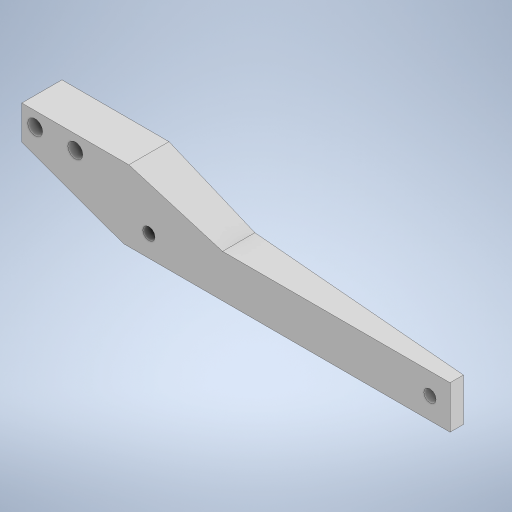
# Autodesk Inventor part: Fan_side_mount
Saved by Autodesk Inventor 2023 (Build 270158000, 158)
## iProperties
Created: 2023-08-19
Part Number: Fan_side_mount
Material: Generic
Document SubType Name: Modeling
Designer: plebbb
Density: 1 g/cm^3
Appearance: Default
Author: plebbb
Autodesk Inventor part; units mm, degrees
ref_plane "YZ Plane" through (0, 0, 0) normal (1, 0, 0) x (0, 1, 0)
ref_plane "XZ Plane" through (0, 0, 0) normal (0, 1, 0) x (-1, 0, 0)
ref_plane "XY Plane" through (0, 0, 0) normal (0, 0, 1) x (1, 0, 0)
sketch "Sketch1" plane through (0, 0, 0) normal (0, 1, 0) x (-1, 0, 0)
  line L0 (0, 0) -> (-40, 0)
  line L1 (-40, 0) -> (-160, 10)
  line L2 (-160, 10) -> (-160, 15)
  line L3 (-160, 15) -> (0, 15)
  line L4 (0, 15) -> (0, 0)
  point P0 (-160, 12.5)
  dimension "d0" = 15
  dimension "d1" = 40
  dimension "d2" = 5
  dimension "d3" = 120
  constraints: 10 end point, 3 perpendicular, 1 horizontal, 1 midpoint
  measures "d0" distance of L3.end L0.start
  measures "d1" distance of L0.start L0.end
  measures "d2" distance of L1.end L2.end
  measures "d3" horizontal distance of L0.end point (-160, 12.5)
extrude "Extrusion1" add sketch "Sketch1" along normal blind 16
sketch "Sketch2" plane through (0, 0, 15) normal (0, 0, 1) x (1, 0, 0)
  circle A0 centre (152.5, 8) radius 2.286
  circle A1 centre (47.5, 8) radius 2.286
  line L0 (160, 0) -> (160, 16) projected
  point P0 (0, 0)
  point P1 (160, 8)
  dimension "d6" = 4.572
  dimension "d7" = 7.5
  dimension "d8" = 105
  constraints: 2 centre point, 2 horizontal alignment, 1 equal radius, 1 midpoint
  measures "d6" diameter of A0
  measures "d7" distance of point (160, 8) A0.centre
  measures "d8" distance of A0.centre A1.centre
extrude "Extrusion2" cut sketch "Sketch2" against normal blind 20
sketch "Sketch3" plane through (40, 0, 0) normal (0, 0, -1) x (-1, 0, 0)
  circle A0 centre (-112.5, 8) radius 2.286 projected
  circle A1 centre (-112.5, 8) radius 6
  circle A2 centre (-7.5, 8) radius 2.286 projected
  circle A3 centre (-7.5, 8) radius 6
  point P0 (40, 0)
  dimension "d11" = 12
  constraints: 2 centre point, 2 coincident, 1 equal radius
  measures "d11" diameter of A1
extrude "Extrusion3" cut sketch "Sketch3" against normal up to surface (10 mm away)
sketch "Sketch4" plane through (40, 0, 0) normal (0, 0, -1) x (-1, 0, 0)
  line L0 (40, 0) -> (40, 16) projected
  line L1 (40, 0) -> (40, 16) projected
  line L2 (40, 16) -> (40, 26.5)
  line L3 (40, 26.5) -> (0, 26.5)
  line L4 (0, 26.5) -> (0, 16)
  line L5 (0, 0) -> (0, 16) projected
  line L6 (0, 0) -> (40, 0) projected
  line L7 (40, 0) -> (40, 16) projected
  line L8 (0, 16) -> (40, 16) projected
  point P0 (40, 8)
  dimension "d14" = 18.5
  constraints: 6 end point, 1 horizontal, 1 midpoint, 1 point on line, 1 vertical
  measures "d14" distance of L2.end point (40, 8)
extrude "Extrusion4" add sketch "Sketch4" against normal up to surface (15 mm away) contours L8 L4 L3 L2
sketch "Sketch5" plane through (40, 0, 0) normal (0, 0, -1) x (-1, 0, 0)
  line L0 (40, 0) -> (-120, 0) projected
  line L1 (2, 0) -> (2, 13.8)
  line L2 (2, 13.8) -> (40, 13.8)
  line L3 (40, 0) -> (40, 26.5) projected
  line L4 (40, 26.5) -> (0, 26.5) projected
  line L5 (0, 26.5) -> (0, 16) projected
  dimension "d17" = 12.7
  dimension "d18" = 2
  constraints: 4 end point, 2 perpendicular, 2 point on line
  measures "d17" distance between parallel lines of L4 L2
  measures "d18" distance between parallel lines of L5 L1
extrude "Extrusion5" cut sketch "Sketch5" against normal through all
sketch "Sketch6" plane through (40, 0, 15) normal (0, 0, -1) x (-1, 0, 0)
  line L0 (40, 13.8) -> (40, 26.5) projected
  line L1 (2, 13.8) -> (2, 0) projected
  line L2 (40, 13.8) -> (2, 0)
  line L3 (2, 13.8) -> (40, 13.8) projected
  point P0 (40, 0)
  constraints: 2 end point
extrude "Extrusion6" add sketch "Sketch6" along normal blind 3
chamfer "Chamfer1" distance 3 angle 45 3 edges at (38, 6.9, 12) (38, 13.8, 6) (19, 13.8, 12)
sketch "Sketch7" plane through (160, 0, 15) normal (0, 0, 1) x (1, 0, 0)
  line L0 (-120, 26.5) -> (-120, 16) projected
  line L1 (-120, 26.5) -> (-85, 16)
  line L2 (-120, 16) -> (0, 16) projected
  point P0 (-160, 0)
  dimension "d29" = 35
  constraints: 2 end point, 1 point on line
  measures "d29" horizontal distance of L0.start L1.end
extrude "Extrusion7" add sketch "Sketch7" against normal up to surface surface through (160, 0, 10) normal (0.0830455, 0, -0.9965458)
sketch "Sketch9" plane through (160, 0, 15) normal (0, 0, 1) x (1, 0, 0)
  circle A0 centre (-140, 21.15) radius 2.794
  circle A1 centre (-155, 21.15) radius 2.794
  line L0 (-160, 13.8) -> (-160, 26.5) projected
  point P0 (-160, 0)
  point P1 (-160, 15.8)
  point P2 (-160, 21.15)
  dimension "d32" = 5.588
  dimension "d33" = 15
  dimension "d34" = 5
  constraints: 2 centre point, 2 horizontal alignment, 1 equal radius, 1 point on line
  measures "d32" diameter of A0
  measures "d33" distance of A0.centre A1.centre
  measures "d34" distance of point (-160, 21.15) A1.centre
extrude "Extrusion8" cut sketch "Sketch9" against normal through all
body "Solid1"
